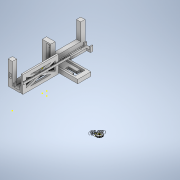
# Autodesk Inventor part: modelGate
Saved by Autodesk Inventor 2020 (Build 240168000, 168)
## iProperties
Created: 2023-10-09
Part Number: modelGate
Material: Generic
Document SubType Name: Sheet Metal
Designer: jirka
Density: 1 g/cm^3
Sheet Metal Rule: Default_mm
Appearance: Default
Author: jirka
Autodesk Inventor part; units mm, degrees
ref_plane "YZ Plane" through (0, 0, 0) normal (1, 0, 0) x (0, 1, 0)
ref_plane "XZ Plane" through (0, 0, 0) normal (0, 1, 0) x (-1, 0, 0)
ref_plane "XY Plane" through (0, 0, 0) normal (0, 0, 1) x (1, 0, 0)
sketch "Sketch1" plane through (0, 0, 0) normal (0, 1, 0) x (-1, 0, 0)
  line L0 (100, 100) -> (-100, 100)
  line L1 (-100, 100) -> (-100, -100)
  line L2 (-100, -100) -> (100, -100)
  line L3 (100, -100) -> (100, 100)
  point P0 (0, 0)
  dimension "d0" = 200
  dimension "d1" = 200
  dimension "d2" = 100
  dimension "d3" = 100
  constraints: 8 end point, 2 parallel, 1 horizontal, 1 perpendicular
  measures "d0" distance of L2.end L0.start
  measures "d1" distance of L1.end L2.end
  measures "d2" distance from line of L2 point (0, 0)
  measures "d3" distance from line of L3 point (0, 0)
extrude "Extrusion1" add sketch "Sketch1" along normal blind 50
sketch "Sketch2" plane through (0, 50, 0) normal (0, 1, 0) x (1, 0, 0)
  line L0 (-100, -100) -> (100, -100) projected
  line L1 (100, 100) -> (-100, 100) projected
  line L2 (0, -100) -> (-20, -100)
  line L3 (-20, -100) -> (-20, 100)
  line L4 (-20, 100) -> (0, 100)
  line L5 (0, 100) -> (0, -100)
  point P0 (0, 0)
  dimension "d6" = 20
  constraints: 8 end point, 2 parallel, 1 horizontal, 1 midpoint, 1 perpendicular, 1 point on line
  measures "d6" distance of L3.end L4.end
extrude "Extrusion2" add sketch "Sketch2" along normal blind 50
sketch "Sketch3" plane through (0, 50, 100) normal (1, 0, 0) x (0, 0, -1)
  line L0 (0, 50) -> (200, 50) projected
  line L1 (0, 50) -> (10, 50)
  line L2 (10, 50) -> (10, 10)
  line L3 (10, 10) -> (0, 10)
  line L4 (0, 10) -> (0, 50)
  line L5 (0, 0) -> (0, 50) projected
  line L6 (10, 10) -> (0, 10)
  line L7 (0, 10) -> (0, 0)
  line L8 (0, 0) -> (10, 0)
  line L9 (10, 0) -> (10, 10)
  line L10 (200, 0) -> (0, 0) projected
  line L11 (10, 50) -> (110, 50)
  line L12 (110, 50) -> (110, 0)
  line L13 (110, 0) -> (10, 0)
  line L14 (10, 0) -> (10, 50)
  line L15 (110, 0) -> (120, 0)
  line L16 (120, 0) -> (120, 50)
  line L17 (120, 50) -> (110, 50)
  line L18 (110, 50) -> (110, 0)
  line L19 (200, 0) -> (200, 50) projected
  line L20 (120, 0) -> (200, 0)
  line L21 (200, 0) -> (200, 10)
  line L22 (200, 10) -> (120, 10)
  line L23 (120, 10) -> (120, 0)
  line L24 (200, 10) -> (190, 10)
  line L25 (190, 10) -> (190, 50)
  line L26 (190, 50) -> (200, 50)
  line L27 (200, 50) -> (200, 10)
  line L28 (10, 0) -> (110, 0)
  line L29 (110, 0) -> (110, 50)
  line L30 (110, 50) -> (10, 50)
  line L31 (10, 50) -> (10, 0)
  line L32 (120, 10) -> (190, 10)
  line L33 (190, 10) -> (190, 50)
  line L34 (190, 50) -> (120, 50)
  line L35 (120, 50) -> (120, 10)
  point P0 (100, -50)
  dimension "d9" = 10
  dimension "d10" = 40
  dimension "d11" = 100
  dimension "d12" = 10
  dimension "d13" = 10
  dimension "d14" = 10
  constraints: 64 end point, 16 parallel, 8 horizontal, 8 perpendicular, 4 point on line
  measures "d9" distance of L2.end L3.end
  measures "d10" distance of L1.end L2.end
  measures "d11" distance of L12.end L13.end
  measures "d12" distance of L17.end L16.end
  measures "d13" distance of L21.end L20.end
  measures "d14" distance of L25.end L26.end
extrude "Extrusion3" cut sketch "Sketch3" against normal blind 34.75 contours L0 L12 L10 L9 L2 | L0 L25 L22 L16
sketch "Sketch4" plane through (0, 100, 0) normal (0, 1, 0) x (1, 0, 0)
  line L0 (100, 100) -> (-100, 100) projected
  line L1 (-20, -100) -> (-10, -100)
  line L2 (-10, -100) -> (-10, 100)
  line L3 (-10, 100) -> (-20, 100)
  line L4 (-20, 100) -> (-20, -100)
  point P0 (0, 0)
  dimension "d17" = 10
  constraints: 8 end point, 2 parallel, 1 horizontal, 1 perpendicular, 1 point on line
  measures "d17" distance of L3.end L2.end
extrude "Extrusion4" cut sketch "Sketch4" against normal blind 50
sketch "Sketch5" plane through (0, 50, -100) normal (1, 0, 0) x (0, 0, -1)
  line L0 (-90, 50) -> (-80, 50) projected
  line L1 (-90, 50) -> (-90, 0) projected
  line L2 (-80, 50) -> (-90, 50)
  line L3 (-90, 50) -> (-90, 3)
  line L4 (-90, 3) -> (-80, 3)
  line L5 (-80, 3) -> (-80, 50)
  line L6 (-80, 10) -> (-80, 50) projected
  line L7 (-90, 50) -> (-80, 50)
  line L8 (-80, 50) -> (-80, 47)
  line L9 (-80, 47) -> (-90, 47)
  line L10 (-90, 47) -> (-90, 50)
  point P0 (-100, -50)
  point P1 (-90, 47)
  point P2 (-80, 47)
  dimension "d20" = 3
  constraints: 16 end point, 4 parallel, 2 horizontal, 2 perpendicular, 2 point on line
  measures "d20" distance of L7.end L8.end
extrude "Extrusion5" add sketch "Sketch5" along normal blind 10 contours L0 L5 L9 L1
sketch "Sketch6" plane through (0, 97, -20) normal (0, -1, 0) x (1, 0, 0)
  line L0 (0, 0) -> (10, 0) projected
  line L1 (10, 10) -> (8, 10)
  line L2 (8, 10) -> (8, 0)
  line L3 (8, 0) -> (10, 0)
  line L4 (10, 0) -> (10, 10)
  point P0 (0, 20)
  constraints: 8 end point, 2 parallel, 1 horizontal, 1 perpendicular, 1 point on line
extrude "Extrusion6" add sketch "Sketch6" along normal blind 47
sketch "Sketch8" plane through (0, 97, -20) normal (0, -1, 0) x (1, 0, 0)
  line L0 (8, 0) -> (8, 10)
  line L1 (0, 10) -> (8, 10)
  line L2 (8, 10) -> (8, 0)
  line L3 (8, 0) -> (0, 0)
  line L4 (0, 0) -> (0, 10)
  line L5 (8, 10) -> (3, 10)
  line L6 (3, 10) -> (3, 7.014316)
  line L7 (3, 7.014316) -> (8, 7.014316)
  line L8 (8, 7.014316) -> (8, 10)
  line L9 (8, 10) -> (5, 10)
  line L10 (5, 10) -> (5, 3.563092)
  line L11 (5, 3.563092) -> (8, 3.563092)
  line L12 (8, 3.563092) -> (8, 10)
  line L13 (0, 0) -> (8, 10)
  line L14 (8, 0) -> (0, 10)
  line L15 (0, 10) -> (1.5, 10)
  line L16 (1.5, 10) -> (1.5, 4.596469)
  line L17 (1.5, 4.596469) -> (0, 4.596469)
  line L18 (0, 4.596469) -> (0, 10)
  line L19 (8, 10) -> (6.5, 10)
  line L20 (6.5, 10) -> (6.5, 3.790614)
  line L21 (6.5, 3.790614) -> (8, 3.790614)
  line L22 (8, 3.790614) -> (8, 10)
  line L23 (4, 5) -> (0.484599, 5)
  line L24 (4, 5) -> (8, 5)
  circle A0 centre (1.5, 5) radius 0.5
  circle A1 centre (6.5, 5) radius 0.5
  point P0 (0, 20)
  dimension "d25" = 3
  dimension "d26" = 1.5
  dimension "d27" = 1.5
  dimension "d28" = 1
  dimension "d29" = 1
  constraints: 48 end point, 10 parallel, 7 horizontal, 5 perpendicular, 5 point on line, 2 centre point, 1 midpoint
  measures "d25" distance of L11.end L10.end
  measures "d26" distance of L16.end L17.end
  measures "d27" distance of L21.end L20.end
  measures "d28" diameter of A0
  measures "d29" diameter of A1
extrude "Extrusion7" add sketch "Sketch8" along normal blind 5 contours A0 L23 L16 L17 | L17 L16 L23 A0 | L23 L16 A0 | A1 L20 L24 | L24 L20 A1 | A1 L24 L20 | A0 L16 L23 | A1 L20 L24
sketch "Sketch9" plane through (6.5, 92, -15) normal (0, -1, 0) x (1, 0, 0)
  circle A0 centre (0, 0) radius 0.75
  circle A1 centre (-5, 0) radius 0.5 projected
  circle A2 centre (-5, 0) radius 0.75
  point P0 (-6.5, 15)
  dimension "d32" = 1.5
  dimension "d33" = 1.5
  constraints: 2 centre point, 1 coincident
  measures "d32" diameter of A0
  measures "d33" diameter of A2
extrude "Extrusion8" add sketch "Sketch9" along normal blind 5 contours A0 | A1 | A2
sketch "Sketch11" plane through (-100, 0, 100) normal (0, 0, 1) x (1, 0, 0)
  line L0 (90, 50) -> (0, 50)
  line L1 (90, 50) -> (110, 50)
  line L2 (110, 50) -> (110, 45)
  line L3 (110, 45) -> (90, 45)
  line L4 (90, 45) -> (90, 50)
  line L5 (0, 50) -> (90, 50)
  line L6 (0, 50) -> (217.198298, 50)
  line L7 (217.198298, 50) -> (217.198298, -19.655801)
  line L8 (217.198298, -19.655801) -> (0, -19.655801)
  line L9 (0, -19.655801) -> (0, 50)
  point P0 (100, 0)
  dimension "d38" = 5
  constraints: 16 end point, 4 parallel, 2 horizontal, 2 perpendicular
  measures "d38" distance of L1.end L2.end
extrude "Extrusion9" cut sketch "Sketch11" against normal blind 379.25 contours L4 L3 L2 L6 L7 L8 L9 L0
sketch "Sketch12" plane through (0, 50, 100) normal (0, 0, 1) x (1, 0, 0)
  line L0 (0, 0) -> (0, 50) projected
  line L1 (10, 50) -> (10, 0) projected
  line L2 (0, 0) -> (10, 0)
  line L3 (10, 0) -> (10, 5)
  line L4 (10, 5) -> (0, 5)
  line L5 (0, 5) -> (0, 0)
  line L6 (10, 0) -> (0, 0) projected
  line L7 (5, 2.5) -> (0, 0)
  line L8 (10, 50) -> (10, 0) projected
  line L9 (5, 2.5) -> (10, 0)
  point P0 (0, -50)
  dimension "d41" = 5
  constraints: 12 end point, 2 parallel, 1 horizontal, 1 perpendicular, 1 point on line
  measures "d41" distance of L3.end L2.end
extrude "Extrusion10" add sketch "Sketch12" against normal up to surface (200 mm away) contours L7 L9 L2
sketch "Sketch13" plane through (0, 50, 0) normal (0, 1, 0) x (1, 0, 0)
  line L0 (-10, -100) -> (0, -100) projected
  line L1 (10, -100) -> (10, 100) projected
  line L2 (0, -100) -> (10, -100)
  line L3 (10, -100) -> (10, -98)
  line L4 (10, -98) -> (0, -98)
  line L5 (0, -98) -> (0, -100)
  point P0 (0, 0)
  constraints: 8 end point, 2 parallel, 1 horizontal, 1 perpendicular, 1 point on line
extrude "Extrusion11" add sketch "Sketch13" along normal blind 5
sketch "Sketch14" plane through (0, 100, 100) normal (1, 0, 0) x (0, 0, -1)
  point P0 (100, -100)
sketch "Sketch15" plane through (0, 50, 0) normal (0, 1, 0) x (1, 0, 0)
  line L0 (0, -90) -> (0, 10) projected
  line L1 (-10, -100) -> (-10, 100) projected
  line L2 (0, 10) -> (-10, 10)
  line L3 (-10, 10) -> (-10, -60)
  line L4 (-10, -60) -> (0, -60)
  line L5 (0, -60) -> (0, 10)
  line L6 (0, -60) -> (-10, -60)
  line L7 (-10, -60) -> (-10, -70)
  line L8 (-10, -70) -> (0, -70)
  line L9 (0, -70) -> (0, -60)
  point P0 (0, 0)
  dimension "d47" = 70
  dimension "d48" = 10
  constraints: 16 end point, 4 parallel, 2 horizontal, 2 perpendicular, 2 point on line
  measures "d47" distance of L3.end L2.end
  measures "d48" distance of L7.end L6.end
extrude "Extrusion12" add sketch "Sketch15" along normal up to surface (50 mm away) contours L8 L1 L4 L0
sketch "Sketch16" plane through (0, 100, 0) normal (0, 1, 0) x (1, 0, 0)
  line L0 (0, -70) -> (-10, -70)
  line L1 (0, -70) -> (-18.634328, -70)
  line L2 (-18.634328, -70) -> (-18.634328, -105.403137)
  line L3 (-18.634328, -105.403137) -> (0, -105.403137)
  line L4 (0, -105.403137) -> (0, -70)
  line L5 (0, -90) -> (0, -70)
  line L6 (0, -70) -> (14.020329, -70)
  line L7 (14.020329, -70) -> (14.020329, -102.468589)
  line L8 (14.020329, -102.468589) -> (0, -102.468589)
  line L9 (0, -102.468589) -> (0, -70)
  point P0 (0, 0)
  constraints: 16 end point, 4 parallel, 2 horizontal, 2 perpendicular
extrude "Extrusion13" cut sketch "Sketch16" against normal blind 80.75
sketch "Sketch17" plane through (0, 50, 0) normal (0, 1, 0) x (1, 0, 0)
  line L0 (10, -70) -> (-10, -70) projected
  line L1 (0, -70) -> (0, -60) projected
  line L2 (10, -70) -> (0, -70)
  line L3 (0, -70) -> (0, -68)
  line L4 (0, -68) -> (10, -68)
  line L5 (10, -68) -> (10, -70)
  point P0 (0, 0)
  constraints: 8 end point, 2 parallel, 1 horizontal, 1 perpendicular, 1 point on line
extrude "Extrusion14" add sketch "Sketch17" along normal blind 10
sketch "Sketch18" plane through (0, 50, 0) normal (0, 1, 0) x (1, 0, 0)
  line L0 (10, -70) -> (10, 100) projected
  line L1 (0, 100) -> (0, 10) projected
  line L2 (10, 100) -> (0, 100)
  line L3 (0, 100) -> (0, 98)
  line L4 (0, 98) -> (10, 98)
  line L5 (10, 98) -> (10, 100)
  point P0 (0, 0)
  constraints: 8 end point, 2 parallel, 1 horizontal, 1 perpendicular, 1 point on line
extrude "Extrusion15" add sketch "Sketch18" along normal blind 10
sketch "Sketch19" plane through (10, 50, -100) normal (1, 0, 0) x (0, 0, -1)
  point P0 (-100, -50)
sketch "Sketch20" plane through (10, 50, -100) normal (1, 0, 0) x (0, 0, -1)
  line L0 (-170, -5) -> (0, -5)
  line L1 (-168, 0) -> (-90, 0)
  line L2 (-170, -5) -> (-139.361866, -5)
  line L3 (-139.361866, -5) -> (-139.361866, 0)
  line L4 (-139.361866, 0) -> (-170, 0)
  line L5 (-170, 0) -> (-170, -5)
  point P0 (-100, -50)
  constraints: 8 end point, 2 parallel, 1 horizontal, 1 perpendicular, 1 point on line
extrude "Extrusion16" add sketch "Sketch20" along normal blind 194.25
sketch "Sketch21" plane through (-10, 50, -10) normal (0, 0, 1) x (1, 0, 0)
  point P0 (10, -50)
sketch "Sketch22" plane through (-10, 100, 70) normal (0, 0, 1) x (1, 0, 0)
  line L0 (214.25, -55) -> (0, -55)
  line L1 (30.72586, -55) -> (34.22586, -55)
  line L2 (34.22586, -55) -> (34.22586, -15)
  line L3 (34.22586, -15) -> (30.72586, -15)
  line L4 (30.72586, -15) -> (30.72586, -55)
  point P0 (10, -100)
  dimension "d59" = 3.5
  dimension "d60" = 40
  constraints: 8 end point, 2 parallel, 1 horizontal, 1 perpendicular, 1 point on line
  measures "d59" distance of L3.end L2.end
  measures "d60" distance of L2.end L1.end
extrude "Extrusion17" add sketch "Sketch22" against normal blind 88
sketch "Sketch23" plane through (-10, 100, 70) normal (0, 0, 1) x (1, 0, 0)
  line L0 (20, -50) -> (20, -55)
  line L1 (20, -50) -> (30.72586, -50)
  line L2 (30.72586, -50) -> (30.72586, -60.1886)
  line L3 (30.72586, -60.1886) -> (20, -60.1886)
  line L4 (20, -60.1886) -> (20, -50)
  line L5 (34.22586, -50) -> (214.25, -50)
  line L6 (34.22586, -50) -> (42.935439, -50)
  line L7 (42.935439, -50) -> (42.935439, -60.1886)
  line L8 (42.935439, -60.1886) -> (34.22586, -60.1886)
  line L9 (34.22586, -60.1886) -> (34.22586, -50)
  point P0 (10, -100)
  constraints: 16 end point, 4 parallel, 2 horizontal, 2 perpendicular
extrude "Extrusion18" cut sketch "Sketch23" against normal blind 88
sketch "Sketch24" plane through (-10, 45, 70) normal (0, 0, 1) x (1, 0, 0)
  line L0 (10, 15) -> (0, 15) projected
  line L1 (20, 5) -> (15, 7.5) projected
  line L2 (10, 15) -> (20, 15)
  line L3 (20, 15) -> (20, 5)
  line L4 (20, 5) -> (10, 5)
  line L5 (10, 5) -> (10, 15)
  point P0 (10, -45)
  constraints: 8 end point, 2 parallel, 1 horizontal, 1 perpendicular
extrude "Extrusion19" cut sketch "Sketch24" against normal blind 175.25
sketch "Sketch25" plane through (-10, 50, -10) normal (0, 0, 1) x (1, 0, 0)
  line L0 (10, 10) -> (10, 47)
  line L1 (10, 47) -> (18, 47)
  line L2 (18, 47) -> (18, -0.008359)
  line L3 (18, -0.008359) -> (10, -0.008359)
  line L4 (10, -0.008359) -> (10, 47)
  line L5 (10, 0) -> (10, 50)
  line L6 (10, 0) -> (12.249984, -0.008359)
  line L7 (12.249984, -0.008359) -> (12.249984, 4.248467)
  line L8 (12.249984, -0.008359) -> (3.49999, -0.008359)
  line L9 (12.249984, -0.008359) -> (15.749984, -0.008359)
  line L10 (15.749984, -0.008359) -> (15.749984, 4.367518)
  line L11 (12.249984, -0.008359) -> (12.249984, 2.991641)
  line L12 (12.249984, 2.991641) -> (15.749984, -0.008359)
  line L13 (12.249984, -0.008359) -> (15.749984, 2.991641)
  line L14 (13.999984, 1.491641) -> (12.249984, 1.491641)
  point P0 (10, -50)
  point P1 (13.999984, 1.491641)
  dimension "d67" = 8
  dimension "d68" = 3.5
  dimension "d69" = 3
  dimension "d80" = 1.5
  constraints: 26 end point, 5 point on line, 3 perpendicular, 2 horizontal, 2 midpoint, 2 parallel
  measures "d67" distance of L2.end L3.end
  measures "d68" distance of L6.end L9.end
  measures "d69" distance of L6.end L11.end
  measures "d80" distance between parallel lines of L9 L14
extrude "Extrusion20" add sketch "Sketch25" along normal up to surface (80 mm away) contours L13 L12 L3
sketch "Sketch28" plane through (-10, 50, -10) normal (0, 0, -1) x (-1, 0, 0)
  line L0 (-15.740233, 0) -> (-13.999984, 1.491641)
  line L1 (-15.740233, 0) -> (-12.259736, 0)
  line L2 (-12.259736, 0) -> (-12.259736, 1.760966)
  line L3 (-12.259736, 1.760966) -> (-15.740233, 1.760966)
  line L4 (-15.740233, 1.760966) -> (-15.740233, 0)
  line L5 (-10, 0) -> (-20, 0)
  line L6 (-15.740233, 0) -> (-13.999984, 1.491641)
  line L7 (-13.999984, 1.491641) -> (-12.259736, 0)
  point P0 (-10, -50)
  constraints: 12 end point, 3 equal length, 1 horizontal, 1 perpendicular, 1 point on line
extrude "Extrusion21" add sketch "Sketch28" along normal up to surface (90 mm away) contours L0 L7 L1
sketch "Sketch31" plane through (8, 60, -10) normal (0, -1, 0) x (1, 0, 0)
  line L0 (0, 0) -> (2, 0) projected
  line L1 (0, -10) -> (2, -10)
  line L2 (2, -10) -> (2, 0)
  line L3 (2, 0) -> (0, 0)
  line L4 (0, 0) -> (0, -10)
  point P0 (-8, 10)
  constraints: 8 end point, 2 parallel, 1 horizontal, 1 perpendicular
extrude "Extrusion24" add sketch "Sketch31" along normal blind 14.25
sketch "Sketch32" plane through (-10, 100, -18) normal (0, 0, -1) x (-1, 0, 0)
  line L0 (-34.22586, -55) -> (-30.72586, -55)
  line L1 (-30.72586, -15) -> (-30.72586, -55)
  line L2 (-34.22586, -55) -> (-30.72586, -55)
  line L3 (-30.72586, -55) -> (-30.72586, -53.5)
  line L4 (-30.72586, -53.5) -> (-34.22586, -53.5)
  line L5 (-34.22586, -53.5) -> (-34.22586, -55)
  line L6 (-34.22586, -53.5) -> (-32.47586, -53.5)
  line L7 (-32.47586, -53.5) -> (-30.72586, -55)
  line L8 (-34.22586, -15) -> (-34.22586, -55)
  line L9 (-32.47586, -53.5) -> (-34.22586, -55)
  point P0 (-10, -100)
  dimension "d81" = 1.5
  constraints: 14 end point, 2 parallel, 1 horizontal, 1 midpoint, 1 perpendicular, 1 point on line
  measures "d81" distance of L3.end L2.end
extrude "Extrusion25" cut sketch "Sketch32" against normal blind 246 contours L9 L7 L0
sketch "Sketch33" plane through (0, 50, 0) normal (0, 1, 0) x (1, 0, 0)
  line L0 (3.999984, -70) -> (3.999984, 100)
  line L1 (3.999984, -70) -> (16.499984, -70)
  line L2 (16.499984, -70) -> (16.499984, -64)
  line L3 (16.499984, -64) -> (3.999984, -64)
  line L4 (3.999984, -64) -> (3.999984, -70)
  line L5 (3.999984, -70) -> (6.099984, -70)
  line L6 (6.099984, -70) -> (6.099984, -64)
  line L7 (6.099984, -64) -> (3.999984, -64)
  line L8 (3.999984, -64) -> (3.999984, -70)
  line L9 (16.499984, -70) -> (14.999984, -70)
  line L10 (14.999984, -64) -> (16.499984, -64)
  line L11 (16.499984, -64) -> (16.499984, -70)
  line L12 (6.099984, -67) -> (7.099984, -67)
  line L13 (14.999984, -67) -> (13.999984, -67)
  line L14 (7.999984, -67) -> (11.999984, -67)
  line L15 (11.999984, -67) -> (12.999984, -67)
  line L16 (3.999984, -70) -> (1.999984, -70)
  line L17 (1.999984, -70) -> (1.999984, -64)
  line L18 (1.999984, -64) -> (3.999984, -64)
  line L19 (3.999984, -64) -> (3.999984, -70)
  line L20 (16.499984, -64) -> (17.999984, -64)
  line L21 (17.999984, -64) -> (17.999984, -70)
  line L22 (17.999984, -70) -> (16.499984, -70)
  line L23 (16.499984, -70) -> (16.499984, -64)
  line L24 (16.499984, -64) -> (14.399984, -64)
  line L25 (14.399984, -64) -> (14.399984, -70)
  line L26 (14.399984, -70) -> (16.499984, -70)
  line L27 (16.499984, -70) -> (16.499984, -64)
  line L28 (14.399984, -67) -> (13.399984, -67)
  circle A0 centre (13.399984, -67) radius 1
  line L29 (6.099984, -67) -> (7.099984, -67)
  circle A1 centre (7.099984, -67) radius 1
  line L30 (8.099984, -67) -> (12.399984, -67)
  point P0 (0, 0)
  dimension "d115" = 2
  dimension "d117" = 2
  dimension "d84" = 12.5
  dimension "d85" = 6
  dimension "d86" = 1
  dimension "d88" = 2.1
  dimension "d90" = 4
  dimension "d91" = 1
  dimension "d113" = 2.1
  dimension "d114" = 1
  dimension "d116" = 1
  dimension "d118" = 4.3
  constraints: 60 end point, 11 parallel, 6 horizontal, 5 perpendicular, 4 point on line, 2 coincident, 2 horizontal alignment, 2 midpoint, 4 other
  measures "d84" distance of L3.end L2.end
  measures "d85" distance of L2.end L1.end
  measures "d86" distance of L12.start L12.end
  measures "d88" distance between parallel lines of L8 L6
  measures "d90" distance of L14.start L14.end
  measures "d91" distance of L14.end L15.end
  measures "d113" distance of L25.end L26.end
  measures "d114" distance of L28.start L28.end
  measures "d116" distance of L12.start L12.end
  measures "d118" distance of L30.start L30.end
extrude "Extrusion26" add sketch "Sketch33" along normal blind 7 contours L16 L17 L18 L0 | A1 | A0 | L2 L20 L21 L22
sketch "Sketch34" plane through (10, 50, -100) normal (1, 0, 0) x (0, 0, -1)
  line L0 (-170, 0) -> (-170, -5) projected
  line L1 (-170, -5) -> (0, -5) projected
  line L2 (-170, 0) -> (-164, 0)
  line L3 (-164, 0) -> (-164, -5)
  line L4 (-164, -5) -> (-170, -5)
  line L5 (-170, -5) -> (-170, 0)
  point P0 (-100, -50)
  dimension "d94" = 6
  constraints: 8 end point, 2 parallel, 1 horizontal, 1 perpendicular, 1 point on line
  measures "d94" distance of L3.end L4.end
extrude "Extrusion27" add sketch "Sketch34" along normal up to surface (7.999984 mm away)
sketch "Sketch35" plane through (0, 50, 0) normal (0, 1, 0) x (1, 0, 0)
  line L0 (3.999984, -64) -> (3.999984, 100)
  line L1 (3.999984, 100) -> (16.499984, 100)
  line L2 (16.499984, 100) -> (16.499984, 94)
  line L3 (16.499984, 94) -> (3.999984, 94)
  line L4 (3.999984, 94) -> (3.999984, 100)
  line L5 (16.499984, 94) -> (14.399984, 94)
  line L6 (14.399984, 94) -> (14.399984, 100)
  line L7 (14.399984, 100) -> (16.499984, 100)
  line L8 (16.499984, 100) -> (16.499984, 94)
  line L9 (16.499984, 97) -> (3.999984, 97)
  line L10 (5.740233, 100) -> (10, 100)
  line L11 (3.999984, 94) -> (6.099984, 94)
  line L12 (6.099984, 94) -> (6.099984, 100)
  line L13 (6.099984, 100) -> (3.999984, 100)
  line L14 (3.999984, 100) -> (3.999984, 94)
  line L15 (6.099984, 97) -> (7.899984, 97)
  line L16 (14.399984, 97) -> (12.499984, 97)
  line L17 (14.399984, 97) -> (13.399984, 97)
  circle A0 centre (13.399984, 97) radius 1
  line L18 (6.099984, 97) -> (7.099984, 97)
  circle A1 centre (7.099984, 97) radius 1
  line L19 (3.999984, 100) -> (1.999984, 100)
  line L20 (1.999984, 100) -> (1.999984, 94)
  line L21 (1.999984, 94) -> (3.999984, 94)
  line L22 (3.999984, 94) -> (3.999984, 100)
  line L23 (16.499984, 94) -> (18.499984, 94)
  line L24 (18.499984, 94) -> (18.499984, 100)
  line L25 (18.499984, 100) -> (16.499984, 100)
  line L26 (16.499984, 100) -> (16.499984, 94)
  point P0 (0, 0)
  dimension "d97" = 12.5
  dimension "d98" = 6
  dimension "d100" = 2.1
  dimension "d101" = 2.1
  dimension "d102" = 1
  dimension "d103" = 2
  dimension "d104" = 1
  dimension "d105" = 2
  constraints: 50 end point, 10 parallel, 7 point on line, 5 horizontal, 5 perpendicular, 4 midpoint, 2 centre point, 2 coincident
  measures "d97" distance of L2.end L3.end
  measures "d98" distance of L1.end L2.end
  measures "d100" distance of L6.end L7.end
  measures "d101" distance between parallel lines of L0 L12
  measures "d102" distance of L16.start L17.end
  measures "d103" diameter of A0
  measures "d104" distance of L15.start L18.end
  measures "d105" diameter of A1
extrude "Extrusion28" add sketch "Sketch35" along normal blind 7 contours L21 L20 L19 L0 | A1 L9 | L9 A1 | L2 L25 L24 L23 | A0 L9 | L9 A0
sketch "Sketch36" plane through (10, 50, -100) normal (1, 0, 0) x (0, 0, -1)
  line L0 (-164, -5) -> (0, -5) projected
  line L1 (0, 0) -> (-80, 0) projected
  line L2 (0, -5) -> (-6, -5)
  line L3 (-6, -5) -> (-6, 0)
  line L4 (-6, 0) -> (0, 0)
  line L5 (0, 0) -> (0, -5)
  point P0 (-100, -50)
  point P1 (-6, -5)
  dimension "d108" = 6
  constraints: 8 end point, 2 parallel, 1 horizontal, 1 perpendicular, 1 point on line
  measures "d108" distance of L3.end L4.end
extrude "Extrusion29" add sketch "Sketch36" along normal up to surface (8.499984 mm away)
sketch "Sketch38" plane through (24.22586, 85, 70) normal (1, 0, 0) x (0, 0, -1)
  line L0 (0, -40) -> (0, 0) projected
  line L1 (88, -40) -> (0, -40) projected
  line L2 (0, 0) -> (84, 0)
  line L3 (84, 0) -> (84, -40)
  line L4 (84, -40) -> (0, -40)
  line L5 (0, -40) -> (0, 0)
  line L6 (88, 0) -> (88, -40) projected
  line L7 (84, -40) -> (88, -40)
  line L8 (88, -40) -> (88, 0)
  line L9 (88, 0) -> (84, 0)
  line L10 (84, 0) -> (84, -40)
  point P0 (70, -85)
  dimension "d119" = 84
  constraints: 16 end point, 4 parallel, 2 horizontal, 2 perpendicular, 1 point on line
  measures "d119" distance of L3.end L4.end
extrude "Extrusion30" cut sketch "Sketch38" against normal blind 9.25 contours L3 L9 L6 L1
sketch "Sketch39" plane through (0, 50, 60) normal (0, 0, -1) x (-1, 0, 0)
  line L0 (10, 0) -> (10, 50)
  line L1 (10, 13.634313) -> (7.6, 13.634313)
  line L2 (7.6, 13.634313) -> (7.6, 18.456327)
  line L3 (7.6, 18.456327) -> (10, 18.456327)
  line L4 (10, 18.456327) -> (10, 13.634313)
  line L5 (7.6, 13.634313) -> (2.5, 13.634313)
  line L6 (2.5, 13.634313) -> (2.5, 23.734313)
  line L7 (2.5, 23.734313) -> (7.6, 23.734313)
  line L8 (7.6, 23.734313) -> (7.6, 13.634313)
  point P0 (0, -50)
  dimension "d122" = 5.1
  dimension "d123" = 10.1
  constraints: 16 end point, 4 parallel, 2 horizontal, 2 perpendicular, 1 point on line
  measures "d122" distance of L6.end L7.end
  measures "d123" distance of L5.end L6.end
extrude "Extrusion31" cut sketch "Sketch39" against normal blind 24.5 contours L5 L6 L7 L8 L2
sketch "Sketch40" plane through (204.25, 50, 70) normal (0, 1, 0) x (1, 0, 0)
  line L0 (0, 0) -> (-171.314561, 0)
  line L1 (0, 0) -> (-7, 0)
  line L2 (-7, 0) -> (-7, 5)
  line L3 (-7, 5) -> (0, 5)
  line L4 (0, 5) -> (0, 0)
  line L5 (0, 5) -> (-7, 0)
  line L6 (-7, 5) -> (0, 0)
  circle A0 centre (-3.5, 2.5) radius 6
  line L7 (-3.5, -3.5) -> (0.194613, -3.5) construction
  line L8 (-9.5, 2.5) -> (-5.805387, 2.5) construction
  line L9 (-3.5, 2.5) -> (-3.5, -7.642392)
  line L10 (0, 0) -> (-3.5, -6.5)
  line L11 (-7, 0) -> (-3.5, -6.5)
  point P0 (-204.25, 70)
  point P1 (-7, 0)
  constraints: 22 end point, 3 horizontal, 2 parallel, 2 point on circle, 1 centre point, 1 coincident, 1 midpoint, 1 perpendicular, 1 point on line, 1 vertical
extrude "Extrusion32" add sketch "Sketch40" along normal blind 24.5 contours L10 A0 L9 L0 | L4 L3 L2 L0 A0 L10 | L9 A0 L11 L0 | L11 A0 L0
sketch "Sketch41" plane through (200.75, 74.5, 67.5) normal (0, 1, 0) x (1, 0, 0)
  arc A0 (-5.454356, -2.5) -> (3.5, 4.873397) centre (0, 0) ccw
  line L0 (0, -6) -> (0, -7)
  line L1 (0, -7) -> (1.335899, -5.407937)
  line L2 (0, -7) -> (2.078291, -7) construction
  line L3 (0, -7) -> (-1.443295, -5.279948)
  line L4 (0, -7) -> (2.245368, -7) construction
  circle A1 centre (0, 0) radius 6
  arc A2 (-0.41955, -6.5) -> (0.41955, -6.5) centre (0, -6.228011) ccw
  point P0 (-200.75, 67.5)
  point P1 (-0.895488, -5.932799)
  point P2 (0.895488, -5.932799)
  point P3 (-0.340711, -6.593957)
  point P4 (0.340711, -6.593957)
  dimension "d135" = 1
  dimension "d136" = 50
  dimension "d137" = 130
  dimension "d184" = 0.5
  constraints: 10 end point, 3 point on circle, 2 equal length, 2 horizontal, 2 point on line, 1 centre point, 1 coincident, 1 vertical, 1 vertical alignment, 2 other
  measures "d135" distance of L0.start L0.end
  measures "d136" angle of L2 L1
  measures "d137" angle of L4 L3
  measures "d184" radius of A2
extrude "Extrusion33" add sketch "Sketch41" against normal up to surface (24.5 mm away) contours L3 A0 L0 A2 | L1 A2 L0 A0
pattern_circular "Circular Pattern1" count 21 over 360 about axis through (200.75, 50, 67.5) along (0, 1, 0) of "Extrusion33"
sketch "Sketch42" plane through (204.25, 50, -100) normal (1, 0, 0) x (0, 0, -1)
  line L0 (-170, 0) -> (-160, 0)
  line L1 (-170, 0) -> (-157.087395, 0)
  line L2 (-157.087395, 0) -> (-157.087395, 2)
  line L3 (-157.087395, 2) -> (-170, 2)
  line L4 (-170, 2) -> (-170, 0)
  line L5 (-170, 0) -> (-170, 7)
  line L6 (-170, 0) -> (-175.773045, 0)
  line L7 (-175.773045, 0) -> (-175.773045, 2)
  line L8 (-175.773045, 2) -> (-170, 2)
  line L9 (-170, 2) -> (-170, 0)
  line L10 (-175.773045, 2) -> (-157.087395, 2)
  line L11 (-157.087395, 2) -> (-157.087395, 24.975118)
  line L12 (-157.087395, 24.975118) -> (-175.773045, 24.975118)
  line L13 (-175.773045, 24.975118) -> (-175.773045, 2)
  point P0 (-100, -50)
  point P1 (-157.087395, 2)
  point P2 (-170, 2)
  constraints: 24 end point, 6 parallel, 3 horizontal, 3 perpendicular, 1 point on line
extrude "Extrusion34" cut sketch "Sketch42" along normal mid plane 24.5 contours L8 L13 L12 L11 L3
sketch "Sketch43" plane through (32.935439, 50, 39.361866) normal (0, 1, 0) x (1, 0, 0)
  line L0 (171.314561, -30.638134) -> (0, -30.638134)
  line L1 (171.314561, -30.638134) -> (171.314561, 0)
  line L2 (0, -30.638134) -> (171.314561, -30.638134)
  line L3 (171.314561, -30.638134) -> (171.314561, 0)
  line L4 (171.314561, 0) -> (0, 0)
  line L5 (0, 0) -> (0, -30.638134)
  point P0 (-32.935439, 39.361866)
  constraints: 8 end point, 2 parallel, 1 horizontal, 1 perpendicular
extrude "Extrusion35" cut sketch "Sketch43" against normal blind 26
sketch "Sketch44" plane through (0, 50, 0) normal (0, 1, 0) x (1, 0, 0)
  point P0 (0, 0)
sketch "Sketch45" plane through (24.22586, 45, 70) normal (1, 0, 0) x (0, 0, -1)
  line L0 (84, 40) -> (84, 0) projected
  line L1 (84, 40) -> (76, 40)
  line L2 (76, 40) -> (76, 32)
  line L3 (76, 32) -> (84, 32)
  line L4 (84, 32) -> (84, 40)
  line L5 (0, 0) -> (84, 0) projected
  line L6 (0, 0) -> (8, 0)
  line L7 (8, 0) -> (8, 8)
  line L8 (8, 8) -> (0, 8)
  line L9 (0, 8) -> (0, 0)
  line L10 (8, 8) -> (76, 8)
  line L11 (76, 8) -> (76, 32)
  line L12 (76, 32) -> (8, 32)
  line L13 (8, 32) -> (8, 8)
  line L14 (4, 5) -> (4, 12) projected
  line L15 (4, 8) -> (76, 36)
  line L16 (80, 55) -> (80, 5) projected
  line L17 (80, 32) -> (8, 4)
  line L18 (0, 0) -> (0, 55) projected
  line L19 (8, 32) -> (0, 32)
  line L20 (0, 32) -> (0, 40)
  line L21 (0, 40) -> (8, 40)
  line L22 (8, 40) -> (8, 32)
  line L23 (84, 0) -> (76, 0)
  line L24 (76, 0) -> (76, 8)
  line L25 (76, 8) -> (84, 8)
  line L26 (84, 8) -> (84, 0)
  line L27 (76, 4) -> (4, 32)
  line L28 (8, 36) -> (80, 8)
  point P0 (70, -45)
  point P1 (65.714286, 8)
  point P2 (42, 17.222222)
  point P3 (18.285714, 8)
  point P4 (49.142857, 20)
  point P5 (76, 9.555556)
  point P6 (76, 30.444444)
  point P7 (18.285714, 32)
  point P8 (42, 22.777778)
  point P9 (65.714286, 32)
  point P10 (34.857143, 20)
  point P11 (8, 30.444444)
  point P12 (8, 9.555556)
  dimension "d147" = 8
  dimension "d148" = 8
  dimension "d149" = 8
  dimension "d150" = 8
  constraints: 48 end point, 10 parallel, 8 midpoint, 5 horizontal, 5 perpendicular, 3 point on line
  measures "d147" distance of L3.end L2.end
  measures "d148" distance of L2.end L1.end
  measures "d149" distance of L8.end L7.end
  measures "d150" distance of L7.end L6.end
extrude "Extrusion36" cut sketch "Sketch45" against normal blind 4.5 contours L11 L28 L17 | L15 L28 L12 | L10 L17 L27 | L15 L13 L27
sketch "Sketch46" plane through (10, 50, -100) normal (1, 0, 0) x (0, 0, -1)
  line L0 (-80, 47) -> (-80, 0) projected
  line L1 (-164, -5) -> (-6, -5) projected
  line L2 (-80, 0) -> (-57, 0)
  line L3 (-57, 0) -> (-57, -5)
  line L4 (-57, -5) -> (-80, -5)
  line L5 (-80, -5) -> (-80, 0)
  point P0 (-100, -50)
  constraints: 8 end point, 2 parallel, 1 horizontal, 1 perpendicular, 1 point on line
extrude "Extrusion37" add sketch "Sketch46" along normal blind 45
sketch "Sketch49" plane through (0, 50, 0) normal (0, 1, 0) x (1, 0, 0)
  line L0 (10, 20) -> (55, 20)
  line L1 (10, 43) -> (55, 43)
  line L2 (10, 20) -> (26, 20)
  line L3 (26, 20) -> (26, 43)
  line L4 (26, 43) -> (10, 43)
  line L5 (10, 43) -> (10, 20)
  line L6 (26, 20) -> (46, 20)
  line L7 (46, 20) -> (46, 28)
  line L8 (46, 28) -> (26, 28)
  line L9 (26, 28) -> (26, 20)
  line L10 (26, 43) -> (46, 43)
  line L11 (46, 43) -> (46, 35)
  line L12 (46, 35) -> (26, 35)
  line L13 (26, 35) -> (26, 43)
  line L14 (26, 20) -> (69.02493, 20)
  line L15 (69.02493, 20) -> (69.02493, 57.037052)
  line L16 (69.02493, 57.037052) -> (26, 57.037052)
  line L17 (26, 57.037052) -> (26, 20)
  point P0 (0, 0)
  dimension "d159" = 16
  dimension "d160" = 8
  dimension "d161" = 8
  constraints: 32 end point, 8 parallel, 4 horizontal, 4 perpendicular, 1 point on line
  measures "d159" distance of L4.end L3.end
  measures "d160" distance of L10.end L11.end
  measures "d161" distance of L6.end L7.end
extrude "Extrusion40" cut sketch "Sketch49" against normal blind 30.5 contours L7 L8 L3 L12 L11 L1 L17 L16 L15 L14 L0
sketch "Sketch50" plane through (0, 50, 0) normal (0, 1, 0) x (1, 0, 0)
  line L0 (10, 20) -> (46, 20) projected
  line L1 (46, 20) -> (56.9, 20)
  line L2 (56.9, 20) -> (56.9, 43)
  line L3 (56.9, 43) -> (46, 43)
  line L4 (46, 43) -> (46, 20)
  line L5 (56.9, 20) -> (66.9, 20)
  line L6 (66.9, 20) -> (66.9, 43)
  line L7 (66.9, 43) -> (56.9, 43)
  line L8 (56.9, 43) -> (56.9, 20)
  point P0 (0, 0)
  dimension "d164" = 10.9
  dimension "d165" = 23
  dimension "d166" = 10
  constraints: 16 end point, 4 parallel, 2 horizontal, 2 perpendicular
  measures "d164" distance of L3.end L2.end
  measures "d165" distance of L2.end L1.end
  measures "d166" distance of L7.end L6.end
extrude "Extrusion41" add sketch "Sketch50" against normal up to surface (5 mm away) contours L2 L7 L6 L5
sketch "Sketch51" plane through (0, 50, 0) normal (0, 1, 0) x (1, 0, 0)
  line L0 (56.9, 43) -> (56.9, 20) projected
  line L1 (66.9, 43) -> (66.9, 20) projected
  line L2 (56.9, 20) -> (66.9, 20)
  line L3 (66.9, 20) -> (66.9, 43)
  line L4 (66.9, 43) -> (56.9, 43)
  line L5 (56.9, 43) -> (56.9, 20)
  point P0 (0, 0)
  constraints: 8 end point, 2 parallel, 1 horizontal, 1 perpendicular
extrude "Extrusion42" add sketch "Sketch51" along normal blind 4
sketch "Sketch52" plane through (0, 50, 0) normal (0, 1, 0) x (1, 0, 0)
  line L0 (10, -64) -> (10, 20) projected
  line L1 (10, 20) -> (66.9, 20)
  line L2 (66.9, 20) -> (66.9, 16)
  line L3 (66.9, 16) -> (10, 16)
  line L4 (10, 16) -> (10, 20)
  line L5 (56.9, 43) -> (66.9, 43) projected
  line L6 (10, 94) -> (10, 43) projected
  line L7 (66.9, 43) -> (10, 43)
  line L8 (10, 43) -> (10, 47)
  line L9 (10, 47) -> (66.9, 47)
  line L10 (66.9, 47) -> (66.9, 43)
  point P0 (0, 0)
  dimension "d171" = 4
  dimension "d172" = 4
  constraints: 16 end point, 4 parallel, 2 horizontal, 2 perpendicular, 1 point on line
  measures "d171" distance of L1.end L2.end
  measures "d172" distance of L7.end L8.end
extrude "Extrusion43" add sketch "Sketch52" along normal blind 4
sketch "Sketch53" plane through (0, 50, 0) normal (0, -1, 0) x (1, 0, 0)
  line L0 (10, -16) -> (66.9, -16) projected
  line L1 (56.9, -20) -> (10, -20) projected
  line L2 (66.9, -16) -> (10, -16)
  line L3 (10, -16) -> (10, -20)
  line L4 (10, -20) -> (66.9, -20)
  line L5 (66.9, -20) -> (66.9, -16)
  line L6 (66.9, -47) -> (10, -47) projected
  line L7 (10, -43) -> (46, -43) projected
  line L8 (66.9, -47) -> (10, -47)
  line L9 (10, -47) -> (10, -43)
  line L10 (10, -43) -> (66.9, -43)
  line L11 (66.9, -43) -> (66.9, -47)
  point P0 (0, 0)
  constraints: 16 end point, 4 parallel, 2 horizontal, 2 perpendicular
extrude "Extrusion44" add sketch "Sketch53" along normal up to surface (5 mm away)
sketch "Sketch56" plane through (0, 50, 0) normal (0, 1, 0) x (1, 0, 0)
  line L0 (3.999984, -64) -> (1.999984, -64)
  line L1 (16.499984, -70) -> (5.740233, -70)
  line L2 (3.999984, -64) -> (6.065704, -64)
  line L3 (6.065704, -64) -> (6.065704, -70)
  line L4 (6.065704, -70) -> (3.999984, -70)
  line L5 (3.999984, -70) -> (3.999984, -64)
  line L6 (3.999984, 94) -> (3.999984, 100)
  line L7 (3.999984, 100) -> (5.892719, 100)
  line L8 (5.892719, 100) -> (5.892719, 94)
  line L9 (5.892719, 94) -> (3.999984, 94)
  line L10 (3.999984, 94) -> (3.999984, 100)
  line L11 (3.999984, -64) -> (3.999984, 94)
  line L12 (3.999984, -64) -> (6.065704, -64)
  line L13 (6.065704, -64) -> (6.065704, -56)
  line L14 (6.065704, -56) -> (3.999984, -56)
  line L15 (3.999984, -56) -> (3.999984, -64)
  line L16 (3.999984, 94) -> (5.892719, 94)
  line L17 (5.892719, 94) -> (5.892719, 86)
  line L18 (5.892719, 86) -> (3.999984, 86)
  line L19 (3.999984, 86) -> (3.999984, 94)
  point P0 (0, 0)
  dimension "d179" = 6
  dimension "d180" = 8
  dimension "d181" = 8
  constraints: 32 end point, 8 parallel, 4 horizontal, 4 perpendicular, 1 point on line
  measures "d179" distance between parallel lines of L4 L2
  measures "d180" distance of L13.end L12.end
  measures "d181" distance of L16.end L17.end
extrude "Extrusion45" cut sketch "Sketch56" along normal blind 10
sketch "Sketch57" plane through (0, 50, 0) normal (0, 1, 0) x (1, 0, 0)
  line L0 (10, 47) -> (10, 43)
  line L1 (8, 20) -> (8, 10)
  line L2 (10, 47) -> (8, 47)
  line L3 (8, 47) -> (8, 15.970911)
  line L4 (8, 15.970911) -> (10, 15.970911)
  line L5 (10, 15.970911) -> (10, 47)
  point P0 (0, 0)
  constraints: 8 end point, 2 parallel, 1 horizontal, 1 perpendicular, 1 point on line
extrude "Extrusion46" add sketch "Sketch57" along normal blind 2
sketch "Sketch58" plane through (200.75, 52, 73.728011) normal (0, 1, 0) x (1, 0, 0)
  line L0 (-5.197107, 3.22746) -> (-6.013666, 3.501809)
  line L1 (-5.367793, 2.383125) -> (-5.197107, 3.22746)
  point P0 (-200.75, 73.728011)
  dimension "d185" = 97.1429
  measures "d185" angle of L0 L1
sketch "Sketch59" plane through (0, 50, 0) normal (0, 1, 0) x (1, 0, 0)
  line L0 (204.25, -65) -> (197.25, -65)
  line L1 (197.25, -70) -> (204.25, -65)
  line L2 (204.25, -65) -> (204.25, -70)
  line L3 (197.25, -65) -> (197.25, -70)
  line L4 (204.25, -70) -> (197.25, -65)
  line L5 (200.75, -67.5) -> (200.593257, -66.414943)
  arc A0 (194.14902, -67.653009) -> (194.199943, -68.332525) centre (194.539404, -67.96542) ccw
  line L6 (194.039404, -67.96542) -> (192.810227, -67.96542)
  line L7 (194.039404, -67.96542) -> (196.242362, -67.96542)
  circle A1 centre (200.75, -67.5) radius 6.726717
  line L8 (194.765679, -67.051537) -> (194.245552, -66.364875)
  circle A2 centre (200.75, -67.5) radius 6.001102
  circle A3 centre (200.75, -67.5) radius 6.001102
  arc A4 (195.382207, -71.344886) -> (195.807067, -71.877643) centre (195.880745, -71.383101) ccw
  line L9 (195.880745, -71.383101) -> (195.514219, -71.723188)
  arc A5 (194.487383, -69.591884) -> (194.736334, -70.226202) centre (194.952508, -69.775348) ccw
  line L10 (194.952508, -69.775348) -> (194.502024, -69.99229)
  line L11 (195.382207, -71.344886) -> (195.552893, -70.500551)
  line L12 (195.382207, -71.344886) -> (195.212297, -72.185384)
  line L13 (196.668214, -71.899119) -> (195.807067, -71.877643)
  line L14 (195.807067, -71.877643) -> (194.857475, -71.853962)
  line L15 (194.487383, -69.591884) -> (194.899358, -68.835371)
  line L16 (194.487383, -69.591884) -> (193.95206, -70.616356)
  line L17 (194.736334, -70.226202) -> (194.005708, -69.99229)
  line L18 (195.27718, -71.864429) -> (194.239111, -70.067014)
  line L19 (195.552893, -70.500551) -> (194.736334, -70.226202)
  line L20 (194.736334, -70.226202) -> (194.887206, -69.777155)
  line L21 (195.552893, -70.500551) -> (195.703765, -70.051504)
  line L22 (195.382207, -71.344886) -> (195.743534, -71.41793)
  line L23 (195.552893, -70.500551) -> (195.91422, -70.573595)
  line L24 (195.382207, -71.344886) -> (194.736334, -70.226202)
  line L25 (196.668214, -71.899119) -> (195.552893, -70.500551)
  line L26 (196.110554, -71.199835) -> (195.27718, -71.864429)
  point P0 (0, 0)
  dimension "d187" = 0.5
  dimension "d188" = 12.0022
  dimension "d189" = 13.45343
  dimension "d194" = 2.07564
  constraints: 38 end point, 7 point on circle, 4 point on line, 3 coincident, 2 centre point, 2 collinear, 2 horizontal, 2 midpoint, 2 perpendicular, 3 other
  measures "d187" radius of A0
  measures "d188" diameter of A2
  measures "d189" diameter of A1
  measures "d194" distance of L18.start L18.end
sketch "Sketch60" plane through (0, 50, 0) normal (0, 1, 0) x (1, 0, 0)
  point P0 (0, 0)
sketch "Sketch61" plane through (24.22586, 45, 70) normal (1, 0, 0) x (0, 0, -1)
  line L0 (0, 0) -> (0, 40) projected
  line L1 (0, 0) -> (111, 0)
  line L2 (111, 0) -> (111, 24.5)
  line L3 (111, 24.5) -> (0, 24.5)
  line L4 (0, 24.5) -> (0, 0)
  line L5 (0, 24.5) -> (111, 24.5)
  line L6 (111, 24.5) -> (111, 20.5)
  line L7 (111, 20.5) -> (0, 20.5)
  line L8 (0, 20.5) -> (0, 24.5)
  point P0 (70, -45)
  point P1 (0, 20.5)
  dimension "d190" = 4
  constraints: 16 end point, 4 parallel, 2 horizontal, 2 perpendicular, 1 point on line
  measures "d190" distance of L5.end L6.end
extrude "Extrusion47" add sketch "Sketch61" along normal blind 2 contours L0 L3 L2 L7
sketch "Sketch62" plane through (24.22586, 85, 70) normal (1, 0, 0) x (0, 0, -1)
  line L0 (0, -15.5) -> (8, -15.5)
  line L1 (0, -15.5) -> (2, -15.5)
  line L2 (2, -15.5) -> (2, -14.05)
  line L3 (2, -14.05) -> (0, -14.05)
  line L4 (0, -14.05) -> (0, -15.5)
  line L5 (1, -14.05) -> (1, -15.5)
  line L6 (111, -15.5) -> (0, -15.5)
  line L7 (0, -15.5) -> (2, -15.5)
  line L8 (2, -15.5) -> (2, -15)
  line L9 (2, -15) -> (0, -15)
  line L10 (0, -15) -> (0, -15.5)
  line L11 (1, -14.05) -> (2, -15)
  line L12 (0, -15) -> (1, -14.05)
  arc A0 (1.375413, -14.406642) -> (0.624587, -14.406642) centre (1, -14.736892) ccw
  point P0 (70, -85)
  point P1 (2, -15.5)
  point P2 (2, -15)
  point P3 (1.310577, -14.345048)
  point P4 (0.689423, -14.345048)
  point P5 (0, -15)
  dimension "d193" = 1.45
  dimension "d195" = 2
  dimension "d206" = 0.5
  dimension "d209" = 0.5
  constraints: 22 end point, 4 parallel, 4 point on line, 3 perpendicular, 2 coincident, 2 horizontal, 2 point on circle, 1 centre point, 1 midpoint
  measures "d193" distance of L2.end L1.end
  measures "d195" distance of L2.end L3.end
  measures "d206" distance of L8.end L7.end
  measures "d209" radius of A0
sketch "Sketch62 outline for Extrusion48" plane through (24.22586, 85, 70) normal (1, 0, 0) x (0, 0, -1)
  line L0 (0, -15.5) -> (2, -15.5)
  line L1 (0, -15) -> (0, -15.5)
  line L2 (0.689423, -14.345048) -> (0, -15)
  arc A0 (1.310577, -14.345048) -> (0.689423, -14.345048) centre (1, -14.736892) ccw
  line L3 (2, -15) -> (1.310577, -14.345048)
  line L4 (2, -15.5) -> (2, -15)
extrude "Extrusion48" add sketch "Sketch62 outline for Extrusion48" along normal blind 2
pattern_linear "Rectangular Pattern1" count 55 spacing 2 along (0, 0, -1) of "Extrusion48"
sketch "Sketch63" plane through (26.22586, 45, 70) normal (1, 0, 0) x (0, 0, -1)
  line L0 (110, 24.5) -> (110, 25) projected
  line L1 (0, 20.5) -> (111, 20.5) projected
  line L2 (110, 24.5) -> (111, 24.5)
  line L3 (111, 24.5) -> (111, 20.5)
  line L4 (111, 20.5) -> (110, 20.5)
  line L5 (110, 20.5) -> (110, 24.5)
  point P0 (70, -45)
  constraints: 8 end point, 2 parallel, 1 horizontal, 1 perpendicular
extrude "Extrusion49" cut sketch "Sketch63" against normal blind 4
sketch "Sketch64" plane through (20.72586, 85, 70) normal (0, 0, 1) x (1, 0, 0)
  point P0 (-20.72586, -85)
sketch "Sketch65" plane through (7.099984, 57, 67) normal (0, 1, 0) x (1, 0, 0)
  line L0 (-1.694133, -2.432299) -> (7.626717, -2.432299)
  line L1 (7.626717, -2.432299) -> (7.626717, 1.956442)
  line L2 (7.626717, 1.956442) -> (-1.694133, 1.956442)
  line L3 (-1.694133, 1.956442) -> (-1.694133, -2.432299)
  line L4 (-1.694133, 161.865052) -> (7.964857, 161.865052)
  line L5 (7.964857, 161.865052) -> (7.964857, 165.701962)
  line L6 (7.964857, 165.701962) -> (-1.694133, 165.701962)
  line L7 (-1.694133, 165.701962) -> (-1.694133, 161.865052)
  point P0 (-7.099984, 67)
  constraints: 16 end point, 4 parallel, 2 horizontal, 2 perpendicular
extrude "Extrusion50" cut sketch "Sketch65" against normal up to surface (7 mm away)
equation "\"d1\" = d0"
equation "\"d2\" = 0.5 * d1"
equation "\"d3\" = 0.5 * d1"
equation "\"BendRadius\" = Thickness"
equation "\"BendReliefWidth\" = Thickness"
equation "\"BendReliefDepth\" = 0.5 * Thickness"
equation "\"CornerReliefSize\" = 4 * Thickness"
equation "\"MinimumRemnant\" = 2 * Thickness"
equation "\"TransitionRadius\" = BendRadius"
equation "\"JacobiRadiusSize\" = BendRadius"
equation "\"GapSize\" = Thickness"
equation "\"Thickness\" = 0.5"
body "Solid1"
